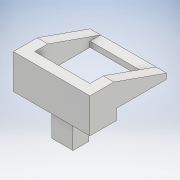
# Autodesk Inventor part: Encoder Mount
Saved by Autodesk Inventor 2018 (Build 220112000, 112)
## iProperties
Created: 2018-01-30
Part Number: Encoder Mount
Material: ABS Plastic
Document SubType Name: Modeling
Designer: Moochster
Density: 1.06 g/cm^3
Appearance: Smooth - White
Author: Moochster
Autodesk Inventor part; units mm, degrees
ref_plane "YZ Plane" through (0, 0, 0) normal (1, 0, 0) x (0, 1, 0)
ref_plane "XZ Plane" through (0, 0, 0) normal (0, 1, 0) x (-1, 0, 0)
sketch "Sketch1" plane through (0, 0, 0) normal (0, 0, 1) x (1, 0, 0)
  line L0 (0, 0) -> (10.4, 0)
  line L1 (10.4, 0) -> (10.4, 10.4)
  line L2 (10.4, 10.4) -> (0, 10.4)
  line L3 (0, 10.4) -> (0, 0)
  line L4 (-2, 12.4) -> (12.4, 12.4)
  line L5 (12.4, 12.4) -> (12.4, -2)
  line L6 (12.4, -2) -> (-2, -2)
  line L7 (-2, -2) -> (-2, 12.4)
  dimension "d0" = 10.4
  dimension "d1" = 10.4
  dimension "d2" = 2
  constraints: 16 end point, 4 parallel, 2 perpendicular, 1 horizontal, 3 other
  measures "d0" distance of L2.end L1.end
  measures "d1" distance of L1.end L0.end
  measures "d2" distance between parallel lines of L2 L4
extrude "Extrusion1" add sketch "Sketch1" along normal blind 1
sketch "Sketch2" plane through (12.4, -2, 0) normal (1, 0, 0) x (0, 0, -1)
  line L0 (0, 14.4) -> (-1, 14.4) projected
  line L1 (-1, 14.4) -> (-4.5, 4.5)
  line L2 (-4.5, 4.5) -> (-4.5, 0)
  line L3 (0, 0) -> (-1, 0) projected
  line L4 (-4.5, 0) -> (-1, 0)
  line L5 (-1, 0) -> (-1, 14.4)
  line L6 (-1, 14.4) -> (-4.5, 14.4)
  line L7 (-4.5, 14.4) -> (-4.5, 4.5)
  point P0 (0, 2)
  dimension "d5" = 4.5
  dimension "d6" = 4.5
  constraints: 12 end point, 3 perpendicular, 1 collinear, 1 horizontal
  measures "d5" distance of L3.start L2.end
  measures "d6" distance of L1.end L2.end
extrude "Extrusion3" add sketch "Sketch2" against normal up to surface (2 mm away) contours L5 L4 L2 L1
ref_plane "Work Plane1" through (5.2, 0, 0) normal (1, 0, 0) x (0, 0, -1)
mirror "Mirror1" about plane through (5.2, 0, 0) normal (1, 0, 0) of "Extrusion3"
sketch "Sketch5" plane through (-2, -2, 0) normal (0, -1, 0) x (1, 0, 0)
  line L0 (14.4, 0) -> (0, 0) projected
  line L1 (14.4, 0) -> (14.4, 4.5) projected
  line L2 (0, 0) -> (14.4, 0)
  line L3 (14.4, 0) -> (14.4, 4.5)
  line L4 (14.4, 4.5) -> (0, 4.5)
  line L5 (0, 4.5) -> (0, 0)
  point P0 (2, 0)
  constraints: 8 end point, 2 parallel, 1 horizontal, 1 perpendicular
extrude "Extrusion4" add sketch "Sketch5" against normal blind 2
sketch "Sketch6" plane through (0, 0, 0) normal (0, 0, -1) x (-1, 0, 0)
  line L0 (-7.2, 3) -> (-3.2, 3)
  line L1 (-3.2, 3) -> (-3.2, 0)
  line L2 (-3.2, 0) -> (-7.2, 0)
  line L3 (-7.2, 0) -> (-7.2, 3)
  line L4 (-12.4, -2) -> (2, -2) projected
  line L5 (-7.2, 3) -> (-12.4, 3)
  line L6 (-3.2, 3) -> (2, 3)
  line L7 (-10.4, -2) -> (0, -2)
  line L8 (-12.4, 3) -> (-12.4, -2)
  line L9 (2, 3) -> (2, -2)
  point P0 (0, 0)
  point P1 (-5.2, 3)
  point P2 (-5.2, -2)
  dimension "d15" = 4
  dimension "d16" = 3
  dimension "d17" = 2
  constraints: 18 end point, 3 point on line, 2 horizontal, 2 midpoint, 2 parallel, 2 vertical, 1 perpendicular, 1 vertical alignment
  measures "d15" distance of L1.end L2.end
  measures "d16" distance of L0.end L1.end
  measures "d17" distance between parallel lines of L4 L2
extrude "Extrusion5" add sketch "Sketch6" along normal blind 8 contours L0 L1 L2 L3
extrude "Extrusion6" add sketch "Sketch6" along normal blind 2 contours L3 L2 L1 L6 L9 L4 L8 L5
sketch "Sketch4" plane through (-2, -2, 0) normal (0, -1, 0) x (1, 0, 0)
  line L0 (14.4, 1) -> (0, 1) projected
  line L1 (0, 1) -> (14.4, 1)
  line L2 (0, 1) -> (0, 4.5)
  line L3 (0, 4.5) -> (2, 4.5)
  line L4 (2, 4.5) -> (2, 3)
  line L5 (2, 3) -> (12.4, 3)
  line L6 (12.4, 3) -> (12.4, 4.5)
  line L7 (12.4, 4.5) -> (14.4, 4.5)
  line L8 (14.4, 4.5) -> (14.4, 1)
  point P0 (2, 0)
  point P1 (12.4, 1)
  point P2 (2, 1)
  dimension "d8" = 2
  constraints: 16 end point, 6 perpendicular, 2 vertical alignment, 1 collinear, 1 point on line, 1 vertical
  measures "d8" distance between parallel lines of L0 L5
body "Solid1"
